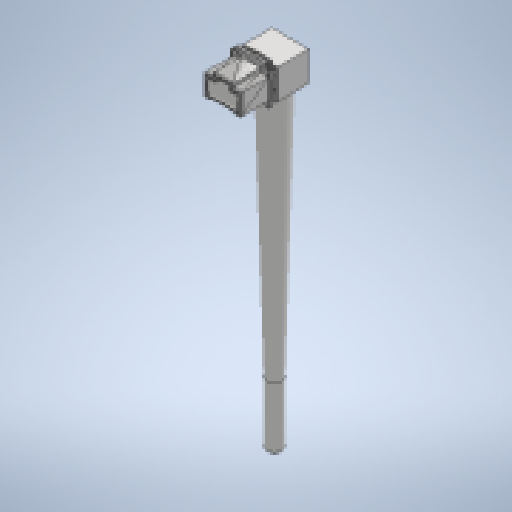
# Autodesk Inventor part: RJ45 Port Cap_Slim
Saved by Autodesk Inventor 2025.1 (Build 291241000, 241)
## iProperties
Created: 2026-04-06
Part Number: RJ45 Port Cap_Slim
Material: Generic
Document SubType Name: Modeling
Designer: User
Density: 1 g/cm^3
Appearance: Default
Author: User
## iProperties of the stored document RJ45 Port Cap_Slim_3DPrint.ipt
Created: 2026-04-06
Part Number: RJ45 Port Cap_Slim_3DPrint
Material: Generic
Document SubType Name: Modeling
Designer: User
Density: 1 g/cm^3
Appearance: Default
Author: User
Autodesk Inventor part; units mm, degrees
ref_plane "YZ Plane" through (0, 0, 0) normal (1, 0, 0) x (0, 1, 0)
ref_plane "XZ Plane" through (0, 0, 0) normal (0, 1, 0) x (-1, 0, 0)
ref_plane "XY Plane" through (0, 0, 0) normal (0, 0, 1) x (1, 0, 0)
sketch "Sketch1" plane through (11.7508, -1.15, -2.5) normal (0, 0, -1) x (-1, 0, 0)
  line L0 (0.2594, -0.35) -> (11.8421, -0.35) projected
  line L1 (11.8421, 9.05) -> (10.9395, 9.05) projected
  line L2 (1.162, 9.05) -> (0.2594, 9.05) projected
  line L3 (11.7508, -0.35) -> (0.2594, -0.35)
  line L4 (0.2594, -0.35) -> (0.2594, 9.05)
  line L5 (0.2594, 9.05) -> (11.7508, 9.05)
  line L6 (11.7508, 9.05) -> (11.7508, -0.35)
  point P0 (11.7508, 1.15)
  constraints: 8 end point, 2 parallel, 1 horizontal, 1 perpendicular, 1 point on line
extrude "Extrusion1" add sketch "Sketch1" along normal blind 10
sketch "Sketch2" plane through (0, -1.5, -2.5) normal (0, -1, 0) x (1, 0, 0)
  line L0 (0, 0) -> (0, -10) projected
  line L1 (11.4914, 0) -> (11.4914, -10) projected
  line L2 (11.4914, -10) -> (0, -10) projected
  line L3 (11.4914, 0) -> (0, 0) projected
  line L4 (0, -10) -> (11.4914, 0)
  circle A0 centre (5.7457, -5) radius 2.5
  point P0 (0, 2.5)
  dimension "d2" = 5
  constraints: 2 end point, 1 centre point, 1 midpoint
  measures "d2" diameter of A0
extrude "Extrusion2" add sketch "Sketch2" along normal blind 100 contours A0 L4 | L4 A0
chamfer "Chamfer1" distance 2 distance2 80 1 edges at (3.2457, -1.5, -7.5) measured on face at (2.7457, -1.5, -7.5)
chamfer "Chamfer2" distance 1 angle 45 1 edges at (3.2457, -101.5, -7.5)
sketch "Sketch3" plane through (11.7508, -1.15, -12.5) normal (0, 0, -1) x (-1, 0, 0)
  line L0 (0.2594, 9.05) -> (0.2594, -0.35) projected
  line L1 (3.0508, 8.8) -> (9.0508, 8.8) projected
  line L2 (11.7508, 7.55) -> (11.7508, -0.85) projected
  line L3 (9.0508, 7.55) -> (11.7508, 7.55) projected
  line L4 (9.0508, 8.8) -> (9.0508, 7.55) projected
  line L5 (3.0508, 7.55) -> (0.3508, 7.55) projected
  line L6 (3.0508, 8.8) -> (3.0508, 7.55) projected
  line L7 (0.3508, 7.55) -> (0.3508, -0.85) projected
  line L8 (0.3508, 1.15) -> (11.7508, 1.15) projected
extrude "Extrusion3" add sketch "Sketch3" against normal blind 20.625
body "Solid1"
